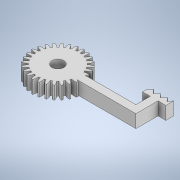
# Autodesk Inventor part: NewConceptArm servo teeth
Saved by Autodesk Inventor 2022 (Build 260153000, 153)
## iProperties
Created: 2022-02-25
Part Number: NewConceptArm servo teeth
Material: Generic
Document SubType Name: Modeling
Designer: Alexa
Density: 1 g/cm^3
Appearance: Default
Author: Alexa
Autodesk Inventor part; units mm, degrees
ref_plane "YZ Plane" through (0, 0, 0) normal (1, 0, 0) x (0, 1, 0)
ref_plane "XZ Plane" through (0, 0, 0) normal (0, 1, 0) x (-1, 0, 0)
ref_plane "XY Plane" through (0, 0, 0) normal (0, 0, 1) x (1, 0, 0)
sketch "Sketch1" plane through (0, 0, 0) normal (0, 1, 0) x (-1, 0, 0)
  circle A0 centre (0, 0) radius 8
  circle A1 centre (0, 0) radius 2
  line L0 (7.9113, 0.5933) -> (7.9113, -0.6067)
  line L1 (9.9113, -0.2567) -> (9.9113, 0.2433)
  line L2 (7.6237, -0.0067) -> (9.0479, -0.0067) construction
  arc A2 (9.9113, 0.2433) -> (7.9113, 0.5933) centre (8.1555, -3.9001) ccw construction
  arc A3 (7.9113, -0.6067) -> (9.9113, -0.2567) centre (8.1555, 3.8866) ccw construction
  arc A4 (9.9113, 0.2433) -> (7.9113, 0.5933) centre (8.1555, -3.9001) ccw construction
  arc A5 (9.9113, 0.2433) -> (7.9777, 0.5964) centre (8.1555, -3.9001) ccw
  arc A6 (7.9767, -0.6098) -> (9.9113, -0.2567) centre (8.1555, 3.8866) ccw
  line L3 (9.4, 0) -> (9.4, -0.4379)
  line L4 (9.4, 0) -> (9.4, 0.4244)
  arc A7 (5.296, -1.8919) -> (5.296, 1.8784) centre (4.6281, -0.0067) ccw
  circle A8 centre (0, 0) radius 8
  dimension "d0" = 16
  dimension "d1" = 4
  dimension "d2" = 0.25
  dimension "d3" = 0.25
  dimension "d4" = 0.6
  dimension "d7" = 1.2
  dimension "d8" = 4.5
  dimension "d10" = 2
  constraints: 18 point on circle, 10 end point, 9 centre point, 4 concentric, 3 coincident, 2 vertical, 1 horizontal, 1 parallel, 1 point on line
  measures "d0" diameter of A0
  measures "d1" diameter of A1
  measures "d2" distance from line of L1.start L2
  measures "d3" distance from line of L1.end L2
  measures "d4" distance from line of L0.start L2
  measures "d7" distance of L0.end L0.start
  measures "d8" radius of A3
  measures "d10" radius of A7
extrude "Extrusion1" add sketch "Sketch1" along normal blind 5
pattern_circular "Circular Pattern1" count 28 over 360 about axis through (0, 0, 0) along (0, 1, 0) of "Extrusion1"
sketch "Sketch8" plane through (0, 5, 0) normal (0, 1, 0) x (1, 0, 0)
  circle A0 centre (0, 0) radius 2.5
  circle A1 centre (0, 0) radius 2
  dimension "d49" = 5
  dimension "d50" = 4
  constraints: 2 centre point, 2 coincident
  measures "d49" diameter of A0
  measures "d50" diameter of A1
extrude "Extrusion6" cut sketch "Sketch8" against normal blind 13.8125
sketch "Sketch9" plane through (0, 5, 0) normal (0, 1, 0) x (1, 0, 0)
  circle A0 centre (0, 0) radius 2.5 projected
  line L0 (0, 0) -> (30, 0)
  line L1 (30, 0) -> (30, -18)
  line L2 (30, -18) -> (0, -18)
  line L3 (0, -18) -> (0, 0)
  circle A1 centre (0, 0) radius 9.5
  circle A2 centre (0, -18) radius 9.5
  line L4 (30, -9) -> (0, -9)
  circle A3 centre (30, -9) radius 2.5
  line L5 (30, 0) -> (5, 0)
  line L6 (5, 0) -> (5, -1.5)
  line L7 (5, -1.5) -> (30, -1.5)
  line L8 (30, -1.5) -> (30, 0)
  line L9 (5, 0) -> (30, 0)
  line L10 (30, 0) -> (30, 1.5)
  line L11 (30, 1.5) -> (5, 1.5)
  line L12 (5, 1.5) -> (5, 0)
  line L13 (30, 1.5) -> (31.5, 1.5)
  line L14 (31.5, 1.5) -> (31.5, -7.5)
  line L15 (31.5, -7.5) -> (30, -7.5)
  line L16 (30, -7.5) -> (30, 1.5)
  line L17 (30, 1.5) -> (28.5, 1.5)
  line L18 (28.5, 1.5) -> (28.5, -7.5)
  line L19 (28.5, -7.5) -> (30, -7.5)
  line L20 (30, -7.5) -> (30, 1.5)
  circle A4 centre (30, -9) radius 1.5
  line L21 (27.5, -9) -> (32.5, -9)
  line L22 (32.5, -9) -> (32.5, -8.5)
  line L23 (32.5, -8.5) -> (27.5, -8.5)
  line L24 (27.5, -8.5) -> (27.5, -9)
  line L25 (28.5, -7.5) -> (27.5, -8.5)
  line L26 (31.5, -7.5) -> (32.5, -8.5)
  line L27 (27.5, -8.5) -> (28.5, -8.5)
  line L28 (32.5, -8.5) -> (31.5, -8.5)
  line L29 (28.5, -7.5) -> (29, -7.5)
  line L30 (31.5, -7.5) -> (31, -7.5)
  line L31 (31, -7.5) -> (31.5, -8.5)
  line L32 (29, -7.5) -> (28.5, -8.5)
  line L33 (5, 1.5) -> (12.096, 1.5)
  line L34 (12.096, 1.5) -> (12.096, -1.5)
  line L35 (12.096, -1.5) -> (5, -1.5)
  line L36 (5, -1.5) -> (5, 1.5)
  dimension "d57" = 5
  dimension "d53" = 30
  dimension "d54" = 18
  dimension "d55" = 19
  dimension "d56" = 19
  dimension "d58" = 25
  dimension "d59" = 1.5
  dimension "d60" = 1.5
  dimension "d61" = 1.5
  dimension "d62" = 9
  dimension "d63" = 1.5
  dimension "d64" = 3
  dimension "d65" = 5
  dimension "d66" = 0.5
  dimension "d67" = 0.5
  dimension "d68" = 0.5
  constraints: 74 end point, 14 parallel, 10 point on line, 7 horizontal, 7 perpendicular, 4 coincident, 3 centre point, 2 midpoint, 1 horizontal alignment, 2 other
  measures "d53" distance of L1.end L2.end
  measures "d54" distance of L0.end L1.end
  measures "d55" diameter of A1
  measures "d56" diameter of A2
  measures "d58" distance of L7.end L6.end
  measures "d59" distance of L6.end L5.end
  measures "d60" distance of L10.end L9.end
  measures "d61" distance of L14.end L15.end
  measures "d62" distance of L13.end L14.end
  measures "d63" distance of L19.end L18.end
  measures "d64" diameter of A4
  measures "d65" distance of L23.end L22.end
  measures "d66" distance of L22.end L21.end
  measures "d67" distance of L18.end L29.end
  measures "d68" distance of L14.end L30.end
extrude "Extrusion7" cut sketch "Sketch9" against normal blind 5 contours L12 L11 A1 L0 | L0 A1 L7 L6 | A1 L11 L34 L0 | L0 L34 L7 A1
sketch "Sketch10" plane through (0, 5, 0) normal (0, 1, 0) x (1, 0, 0)
  circle A0 centre (0, 0) radius 2.5 projected
  line L0 (0, 0) -> (30, 0)
  line L1 (30, 0) -> (30, -9)
  line L2 (30, -9) -> (0, -9)
  line L3 (0, -9) -> (0, 0)
  line L4 (5, 1.5) -> (30, 1.5)
  line L5 (30, 1.5) -> (30, -1.5)
  line L6 (30, -1.5) -> (5, -1.5)
  line L7 (5, -1.5) -> (5, 1.5)
  line L8 (31.5, 1.5) -> (28.5, 1.5)
  line L9 (28.5, 1.5) -> (28.5, -7.5)
  line L10 (28.5, -7.5) -> (31.5, -7.5)
  line L11 (31.5, -7.5) -> (31.5, 1.5)
  circle A1 centre (30, -9) radius 1.5
  circle A2 centre (30, -9) radius 2.5
  line L12 (27.5, -9) -> (32.4495, -9)
  line L13 (32.4495, -9) -> (32.4495, -8.5)
  line L14 (27.5, -8.5) -> (27.5, -9)
  line L15 (27.5, -9) -> (32.5, -9)
  line L16 (32.5, -9) -> (32.5, -8.5)
  line L17 (32.5, -8.5) -> (27.5, -8.5)
  line L18 (27.5, -8.5) -> (27.5, -9)
  line L19 (28.5, -7.5) -> (27.5, -8.5)
  line L20 (31.5, -7.5) -> (32.5, -8.5)
  line L21 (28.5, -7.5) -> (29, -7.5)
  line L22 (31.5, -7.5) -> (31, -7.5)
  line L23 (29, -7.5) -> (28.5, -8.5)
  line L24 (31, -7.5) -> (31.5, -8.5)
  point P0 (28.5, -1.5)
  point P1 (28.5, -7)
  point P2 (27.5505, -8.5)
  point P3 (28.5858, -8.5)
  point P4 (31.4142, -8.5)
  point P5 (31.5, -7)
  dimension "d71" = 30
  dimension "d72" = 9
  dimension "d73" = 3
  dimension "d74" = 3
  dimension "d75" = 9
  dimension "d76" = 3
  dimension "d77" = 5
  dimension "d78" = 0.5
  dimension "d79" = 5
  dimension "d80" = 0.5
  dimension "d81" = 0.5
  constraints: 50 end point, 9 parallel, 7 point on line, 6 perpendicular, 5 horizontal, 2 centre point, 2 coincident, 2 point on circle
  measures "d71" distance of L1.end L2.end
  measures "d72" distance of L0.end L1.end
  measures "d73" distance of L4.end L5.end
  measures "d74" distance of L10.end L9.end
  measures "d75" distance of L9.end L8.end
  measures "d76" diameter of A1
  measures "d77" diameter of A2
  measures "d78" distance of L13.end L12.end
  measures "d79" distance of L17.end L16.end
  measures "d80" distance of L9.end L21.end
  measures "d81" distance of L10.end L22.end
extrude "Extrusion8" add sketch "Sketch10" against normal blind 5 contours L7 L4 L9 L0 | L0 L9 L6 L7 | L9 L4 L5 L0 | L0 L1 L6 L9 | L5 L8 L11 A2 L1 | L6 L1 A2 L9 | A2 L19 L10 L23 L17 | A2 L1 L10 L9 | L9 L19 A2 | L17 L23 L10 A1 | L17 L24 L10 L20 A2 | A2 L11 L10 L1 | L10 L24 L17 A1 | L20 L11 A2
sketch "Sketch11" plane through (0, 5, 0) normal (0, 1, 0) x (1, 0, 0)
  circle A0 centre (0, 0) radius 2.5
  circle A1 centre (0, 0) radius 2.3
  dimension "d84" = 4.6
  constraints: 2 centre point, 2 coincident
  measures "d84" diameter of A1
extrude "Extrusion9" add sketch "Sketch11" against normal blind 5
sketch "Sketch12" plane through (0, 5, 0) normal (0, 1, 0) x (1, 0, 0)
  line L0 (28.5, -1.5) -> (35.444, -1.5)
  line L1 (35.444, -1.5) -> (35.444, -9.6454)
  line L2 (35.444, -9.6454) -> (28.5, -9.6454)
  line L3 (28.5, -9.6454) -> (28.5, -1.5)
  line L4 (35.444, -1.5) -> (25.1031, -1.5)
  line L5 (25.1031, -1.5) -> (25.1031, -9.6454)
  line L6 (25.1031, -9.6454) -> (35.444, -9.6454)
  line L7 (35.444, -9.6454) -> (35.444, -1.5)
  point P0 (0, 0)
  constraints: 16 end point, 4 parallel, 2 horizontal, 2 perpendicular, 1 point on line
extrude "Extrusion10" cut sketch "Sketch12" against normal blind 12.225
sketch "Sketch13" plane through (0, 5, 0) normal (0, 1, 0) x (1, 0, 0)
  line L0 (31.5, -1.5) -> (31.5, 1.5) projected
  line L1 (31.5, 0) -> (28.5, 0)
  line L2 (28.5, 0) -> (28.5, 9)
  line L3 (28.5, 9) -> (31.5, 9)
  line L4 (31.5, 9) -> (31.5, 0)
  line L5 (30, 0) -> (30, 25)
  circle A0 centre (30, 25) radius 15.5
  line L6 (31.5, 9) -> (34.5, 9)
  line L7 (28.5, 9) -> (25.5, 9)
  line L8 (25.5, 9) -> (25.5, 10.1676)
  line L9 (34.5, 9) -> (34.5, 10.1676)
  line L10 (34.5, 9) -> (25.5, 9)
  line L11 (25.5, 9) -> (25.5, 7)
  line L12 (25.5, 7) -> (34.5, 7)
  line L13 (34.5, 7) -> (34.5, 9)
  line L14 (31.5, 1.5) -> (8.9321, 1.5) projected
  line L15 (31.5, 1.5) -> (28.5, 1.5)
  point P0 (0, 0)
  point P1 (28.5, 7)
  point P2 (31.5, 7)
  dimension "d89" = 3
  dimension "d90" = 9
  dimension "d91" = 25
  dimension "d92" = 31
  dimension "d93" = 3
  dimension "d94" = 3
  dimension "d95" = 2
  constraints: 28 end point, 4 horizontal, 4 parallel, 3 perpendicular, 2 midpoint, 2 point on circle, 2 point on line, 1 centre point, 1 coincident, 1 vertical
  measures "d89" distance of L2.end L3.end
  measures "d90" distance of L1.end L2.end
  measures "d91" distance of L5.start L5.end
  measures "d92" diameter of A0
  measures "d93" distance of L3.end L6.end
  measures "d94" distance of L2.end L7.end
  measures "d95" distance of L11.end L10.end
extrude "Extrusion11" add sketch "Sketch13" against normal blind 5 contours L14 L5 L12 L4 | L12 L5 L3 L4 | L4 L6 L13 L12 | L14 L2 L12 L5 | L3 L5 A0 L9 L6 | L12 L2 L3 L5 | L3 L7 L8 A0 L5 | L12 L11 L7 L2
sketch "Sketch14" plane through (0, 5, 0) normal (0, 1, 0) x (1, 0, 0)
  line L0 (25.5, 7) -> (28.5, 7) projected
  line L1 (25.5, 7) -> (27.5, 7)
  line L2 (27.5, 7) -> (27.5, 11.8415)
  line L3 (27.5, 11.8415) -> (25.5, 11.8415)
  line L4 (25.5, 11.8415) -> (25.5, 7)
  line L5 (34.5, 7) -> (31.5, 7) projected
  line L6 (34.5, 7) -> (33.5, 7)
  line L7 (33.5, 7) -> (33.5, 12.9828)
  line L8 (33.5, 12.9828) -> (34.5, 12.9828)
  line L9 (34.5, 12.9828) -> (34.5, 7)
  point P0 (0, 0)
  dimension "d98" = 2
  dimension "d99" = 1
  constraints: 16 end point, 4 parallel, 2 horizontal, 2 perpendicular
  measures "d98" distance of L3.end L2.end
  measures "d99" distance of L7.end L8.end
extrude "Extrusion12" cut sketch "Sketch14" against normal blind 10.6375
sketch "Sketch15" plane through (0, 5, 0) normal (0, 1, 0) x (1, 0, 0)
  line L0 (33.5, 7) -> (33.5, 9.9003) projected
  line L1 (33.5, 7) -> (32.2499, 7)
  line L2 (32.2499, 7) -> (32.2499, 11.5082)
  line L3 (32.2499, 11.5082) -> (33.5, 11.5082)
  line L4 (33.5, 11.5082) -> (33.5, 7)
  line L5 (33.5, 7) -> (32.5, 7)
  line L6 (32.5, 7) -> (32.5, 12.0221)
  line L7 (32.5, 12.0221) -> (33.5, 12.0221)
  line L8 (33.5, 12.0221) -> (33.5, 7)
  line L9 (8.8997, -1.5) -> (31.5, -1.5) projected
  line L10 (28.5, 1.5) -> (27.5, 1.5)
  line L11 (27.5, 1.5) -> (27.5, -1.5)
  line L12 (27.5, -1.5) -> (28.5, -1.5)
  line L13 (28.5, -1.5) -> (28.5, 1.5)
  point P0 (0, 0)
  dimension "d102" = 1
  dimension "d103" = 1
  constraints: 24 end point, 6 parallel, 3 horizontal, 3 perpendicular, 1 point on line
  measures "d102" distance of L6.end L7.end
  measures "d103" distance of L12.end L11.end
extrude "Extrusion13" cut sketch "Sketch15" against normal blind 10 contours L11 L10 L13 L9
sketch "Sketch16" plane through (0, 5, 0) normal (0, 1, 0) x (1, 0, 0)
  line L0 (31.5, 7) -> (31.5, -1.5) projected
  line L1 (28.5, -1.5) -> (28.5, 7) projected
  line L2 (31.5, -1.5) -> (28.5, -1.5)
  line L3 (28.5, -1.5) -> (28.5, 0)
  line L4 (28.5, 0) -> (31.5, 0)
  line L5 (31.5, 0) -> (31.5, -1.5)
  line L6 (31.5, -1.5) -> (28.5, -1.5)
  line L7 (28.5, -1.5) -> (28.5, 7)
  line L8 (28.5, 7) -> (31.5, 7)
  line L9 (31.5, 7) -> (31.5, -1.5)
  line L10 (27.5, -1.5) -> (27.5, 1.5) projected
  line L11 (27.5, -1.5) -> (30.5, -1.5)
  line L12 (30.5, -1.5) -> (30.5, 7)
  line L13 (30.5, 7) -> (27.5, 7)
  line L14 (27.5, 7) -> (27.5, -1.5)
  line L15 (27.5, 0) -> (29, 0)
  line L16 (35.3817, -5.8179) -> (27.164, -5.8179)
  line L17 (27.164, -5.8179) -> (27.164, 12.5544)
  line L18 (27.164, 12.5544) -> (35.3817, 12.5544)
  line L19 (35.3817, 12.5544) -> (35.3817, -5.8179)
  line L20 (27.5, -1.5) -> (34.6587, -1.5)
  line L21 (34.6587, -1.5) -> (34.6587, 10.9327)
  line L22 (34.6587, 10.9327) -> (27.5, 10.9327)
  line L23 (27.5, 10.9327) -> (27.5, -1.5)
  point P0 (0, 0)
  dimension "d106" = 3
  dimension "d107" = 1.5
  constraints: 42 end point, 10 parallel, 5 horizontal, 5 perpendicular, 4 point on line
  measures "d106" distance of L13.end L12.end
  measures "d107" distance of L15.start L15.end
extrude "Extrusion14" cut sketch "Sketch16" against normal blind 15.4 contours L8 L13 L23 L22 L21 L20 L0 | L0 L4 L12 L8 | L0 L2 L12 L4 | L12 L4 L1 L8 | L12 L2 L1 L4
sketch "Sketch17" plane through (0, 5, 0) normal (0, 1, 0) x (1, 0, 0)
  line L0 (27.5, -1.5) -> (8.8997, -1.5) projected
  line L1 (27.5, -1.5) -> (30.5, -1.5)
  line L2 (30.5, -1.5) -> (30.5, 5.5)
  line L3 (30.5, 5.5) -> (27.5, 5.5)
  line L4 (27.5, 5.5) -> (27.5, -1.5)
  line L5 (29, 0) -> (29, 25)
  circle A0 centre (29, 25) radius 15.5
  line L6 (30.5, 5.5) -> (30.5, 9.5728)
  line L7 (27.5, 5.5) -> (27.5, 9.5728)
  line L8 (30.5, 9.5728) -> (32.5, 9.5728)
  line L9 (32.5, 9.5728) -> (32.5, 7.5728)
  line L10 (32.5, 7.5728) -> (30.5, 7.5728)
  line L11 (30.5, 7.5728) -> (30.5, 9.5728)
  line L12 (32.5, 9.5728) -> (32.5, 9.9003)
  line L13 (27.5, 9.5728) -> (26.5, 9.5728)
  line L14 (26.5, 9.5728) -> (26.5, 7.5728)
  line L15 (26.5, 7.5728) -> (27.5, 7.5728)
  line L16 (27.5, 7.5728) -> (27.5, 9.5728)
  line L17 (26.5, 9.5728) -> (26.5, 9.7365)
  point P0 (0, 0)
  point P1 (26.5, 9.7029)
  dimension "d110" = 3
  dimension "d111" = 7
  dimension "d112" = 25
  dimension "d113" = 31
  dimension "d114" = 2
  dimension "d115" = 2
  dimension "d116" = 1
  constraints: 34 end point, 7 parallel, 4 vertical, 3 horizontal, 3 perpendicular, 3 point on circle, 1 centre point, 1 coincident
  measures "d110" distance of L3.end L2.end
  measures "d111" distance of L2.end L1.end
  measures "d112" distance of L5.start L5.end
  measures "d113" diameter of A0
  measures "d114" distance of L9.end L10.end
  measures "d115" distance of L8.end L9.end
  measures "d116" distance of L15.end L14.end
extrude "Extrusion15" add sketch "Sketch17" against normal blind 5 contours L4 L3 L2 L1 | L7 A0 L5 L3 | L3 L5 A0 L6 | L15 L14 L13 L7 | L6 L8 L9 L10 | L13 L17 A0 | A0 L12 L8
sketch "Sketch18" plane through (0, 5, 0) normal (0, 1, 0) x (1, 0, 0)
  line L0 (27.5, 1.5) -> (27.5, 7.5728) projected
  line L1 (27.5, 7.5728) -> (26.0844, 7.5728)
  line L2 (26.0844, 7.5728) -> (26.0844, 11.3347)
  line L3 (26.0844, 11.3347) -> (27.5, 11.3347)
  line L4 (27.5, 11.3347) -> (27.5, 7.5728)
  point P0 (0, 0)
  constraints: 8 end point, 2 parallel, 1 horizontal, 1 perpendicular
extrude "Extrusion16" cut sketch "Sketch18" against normal blind 7.7
sketch "Sketch19" plane through (0, 5, 0) normal (0, 1, 0) x (1, 0, 0)
  line L0 (27.5, 1.5) -> (34.147, 1.5)
  line L1 (34.147, 1.5) -> (34.147, 14.0546)
  line L2 (34.147, 14.0546) -> (27.5, 14.0546)
  line L3 (27.5, 14.0546) -> (27.5, 1.5)
  line L4 (27.5, 1.5) -> (33.2737, 1.5)
  line L5 (33.2737, 1.5) -> (33.2737, -3.2769)
  line L6 (33.2737, -3.2769) -> (27.5, -3.2769)
  line L7 (27.5, -3.2769) -> (27.5, 1.5)
  point P0 (0, 0)
  constraints: 16 end point, 4 parallel, 2 horizontal, 2 perpendicular
extrude "Extrusion17" cut sketch "Sketch19" against normal blind 11.35
sketch "Sketch20" plane through (27.5, 5, 1.5) normal (1, 0, 0) x (0, 0, -1)
  line L0 (0, -5) -> (0, 0) projected
  line L1 (3, 0) -> (3, -5) projected
  line L2 (0, 0) -> (3, 0)
  line L3 (3, 0) -> (3, -5)
  line L4 (3, -5) -> (0, -5)
  line L5 (0, -5) -> (0, 0)
  point P0 (1.5, -5)
  constraints: 8 end point, 2 parallel, 1 horizontal, 1 perpendicular
extrude "Extrusion18" add sketch "Sketch20" along normal blind 1
sketch "Sketch21" plane through (0, 5, 0) normal (0, 1, 0) x (1, 0, 0)
  line L0 (0, 0) -> (30, 0)
  line L1 (30, 0) -> (30, 10)
  line L2 (30, 10) -> (0, 10)
  line L3 (0, 10) -> (0, 0)
  line L4 (28.5, -1.5) -> (8.8997, -1.5) projected
  line L5 (28.5, -1.5) -> (31.5, -1.5)
  line L6 (31.5, -1.5) -> (31.5, 1.5)
  line L7 (31.5, 1.5) -> (28.5, 1.5)
  line L8 (28.5, 1.5) -> (28.5, -1.5)
  line L9 (31.5, 1.5) -> (28.5, 1.5)
  line L10 (28.5, 1.5) -> (28.5, 10)
  line L11 (28.5, 10) -> (31.5, 10)
  line L12 (31.5, 10) -> (31.5, 1.5)
  line L13 (31.5, 10) -> (34.5, 10)
  line L14 (34.5, 10) -> (34.5, 7)
  line L15 (34.5, 7) -> (31.5, 7)
  line L16 (31.5, 7) -> (31.5, 10)
  line L17 (28.5, 10) -> (25.5, 10)
  line L18 (25.5, 10) -> (25.5, 7)
  line L19 (25.5, 7) -> (28.5, 7)
  line L20 (28.5, 7) -> (28.5, 10)
  dimension "d125" = 30
  dimension "d126" = 10
  dimension "d127" = 3
  dimension "d128" = 3
  dimension "d129" = 3
  dimension "d130" = 3
  dimension "d131" = 3
  dimension "d132" = 3
  constraints: 40 end point, 10 parallel, 5 horizontal, 5 perpendicular, 2 point on line
  measures "d125" distance of L2.end L1.end
  measures "d126" distance of L1.end L0.end
  measures "d127" distance of L7.end L6.end
  measures "d128" distance of L6.end L5.end
  measures "d129" distance of L14.end L15.end
  measures "d130" distance of L13.end L14.end
  measures "d131" distance of L19.end L18.end
  measures "d132" distance of L18.end L17.end
extrude "Extrusion19" add sketch "Sketch21" against normal blind 5 contours L8 L7 L1 L0 | L0 L1 L7 L6 L5 L8 | L10 L2 L1 L7 | L2 L10 L19 L18 | L1 L11 L12 L7 | L13 L14 L15 L12
sketch "Sketch22" plane through (0, 5, 0) normal (0, 1, 0) x (1, 0, 0)
  line L0 (34.5, 10) -> (34.5, 7) projected
  line L1 (34.5, 8.5) -> (25.5, 8.5)
  line L2 (25.5, 10) -> (25.5, 7) projected
  line L3 (25.5, 8.5) -> (26.8232, 10)
  line L4 (25.5, 10) -> (34.5, 10) projected
  line L5 (26.8232, 10) -> (28.1461, 8.5)
  line L6 (28.1461, 8.5) -> (29.4693, 10)
  line L7 (29.4693, 10) -> (30.7922, 8.5)
  line L8 (30.7922, 8.5) -> (32.1154, 10)
  line L9 (32.1154, 10) -> (33.4382, 8.5)
  line L10 (33.4382, 8.5) -> (34.5, 10)
  point P0 (0, 0)
  dimension "d135" = 2
  constraints: 16 end point, 4 parallel, 3 point on line, 2 midpoint
  measures "d135" distance of L3.end L5.end
extrude "Extrusion20" cut sketch "Sketch22" against normal blind 14.05 contours L10 L9 L4 | L8 L7 L4 | L6 L5 L4 | L3 L2 L4
body "Solid1"
